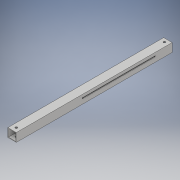
# Autodesk Inventor part: CLB_031_ScissorLiftBase19
Saved by Autodesk Inventor 2018.3 (Build 223284000, 284)
## iProperties
Created: 2020-01-24
Part Number: CLB_031_ScissorLiftBase19
Material: Generic
Document SubType Name: Modeling
Designer: Cooper
Density: 1 g/cm^3
Appearance: Default
Mass: 64.5264 g
Surface Area: 826.986 cm^2
Volume: 64.5264 cm^3
Author: Cooper
Autodesk Inventor part; units mm, degrees
ref_plane "YZ Plane" through (0, 0, 0) normal (1, 0, 0) x (0, 1, 0)
ref_plane "XZ Plane" through (0, 0, 0) normal (0, 1, 0) x (-1, 0, 0)
ref_plane "XY Plane" through (0, 0, 0) normal (0, 0, 1) x (1, 0, 0)
sketch "Sketch1" plane through (0, 0, 0) normal (0, 0, 1) x (1, 0, 0)
  line L0 (0, 0) -> (25.4, 0)
  line L1 (25.4, 0) -> (25.4, 25.4)
  line L2 (25.4, 25.4) -> (0, 25.4)
  line L3 (0, 25.4) -> (0, 0)
  line L4 (1.5875, 23.8125) -> (23.8125, 23.8125)
  line L5 (23.8125, 23.8125) -> (23.8125, 1.5875)
  line L6 (23.8125, 1.5875) -> (1.5875, 1.5875)
  line L7 (1.5875, 1.5875) -> (1.5875, 23.8125)
  dimension "d0" = 25.4
  dimension "d1" = 25.4
  dimension "d2" = 1.5875
  constraints: 16 end point, 4 parallel, 2 perpendicular, 1 horizontal, 3 other
  measures "d0" distance of L2.end L0.start
  measures "d1" distance of L0.start L0.end
  measures "d2" distance between parallel lines of L2 L4
extrude "Extrusion1" add sketch "Sketch1" along normal blind 508
sketch "Sketch2" plane through (0, 0, 0) normal (-1, 0, 0) x (0, 0, 1)
  line L0 (0, 25.4) -> (0, 0) projected
  line L1 (0, 0) -> (508, 0) projected
  line L2 (508, 25.4) -> (508, 0) projected
  line L3 (0, 25.4) -> (508, 25.4) projected
  line L4 (95.25, 16.8275) -> (311.15, 16.8275)
  arc A0 (311.15, 13.6525) -> (311.15, 16.8275) centre (311.15, 15.24) ccw
  line L5 (311.15, 13.6525) -> (95.25, 13.6525)
  arc A1 (95.25, 16.8275) -> (95.25, 13.6525) centre (95.25, 15.24) ccw
  dimension "d5" = 3.175
  dimension "d6" = 215.9
  dimension "d9" = 10.16
  dimension "d24" = 95.25
  constraints: 4 end point, 4 point on circle, 4 tangent, 2 centre point, 1 horizontal, 1 parallel
  measures "d5" distance between parallel lines of L5 L4
  measures "d6" distance of A0.centre A1.centre
  measures "d9" distance from line of L3 A1.centre
  measures "d24" distance from line of L0 A1.centre
extrude "Extrusion2" cut sketch "Sketch2" against normal through all contours L4 A0 L5 A1
sketch "Sketch3" plane through (0, 25.4, 0) normal (0, 1, 0) x (1, 0, 0)
  line L0 (25.4, 0) -> (0, 0) projected
  line L1 (0, 0) -> (0, -508) projected
  line L2 (25.4, -508) -> (0, -508) projected
  line L3 (25.4, 0) -> (25.4, -508) projected
  point P0 (0, 0)
  point P1 (12.7, -495.3)
  dimension "d13" = 12.7
  dimension "d14" = 12.7
  dimension "d23" = 12.7
  measures "d13" distance from line of L1 point (12.7, -495.3)
  measures "d14" distance from line of L3 point (12.7, -495.3)
  measures "d23" distance from line of L2 point (12.7, -495.3)
hole "Hole1" at (12.7, 25.4, 495.3) direction (0, -1, 0) diameter 6.35 end through all
sketch "Sketch4" plane through (0, 0, 0) normal (0, 0, -1) x (-1, 0, 0)
  line L0 (-35.9744, 31.9382) -> (12.1084, 31.9382)
  line L1 (12.1084, 31.9382) -> (12.1084, -6.8439)
  line L2 (12.1084, -6.8439) -> (-35.9744, -6.8439)
  line L3 (-35.9744, -6.8439) -> (-35.9744, 31.9382)
  point P0 (0, 0)
  constraints: 8 end point, 2 parallel, 1 horizontal, 1 perpendicular
extrude "Extrusion3" cut sketch "Sketch4" against normal blind 44.45
sketch "Sketch5" plane through (0, 0, 508) normal (0, -1, 0) x (1, 0, 0)
  line L0 (0, -463.55) -> (25.4, -463.55) projected
  line L1 (25.4, -463.55) -> (25.4, 0) projected
  point P0 (0, -508)
  point P1 (12.7, -453.39)
  dimension "d27" = 10.16
  dimension "d28" = 12.7
  measures "d27" distance from line of L0 point (12.7, -453.39)
  measures "d28" distance from line of L1 point (12.7, -453.39)
hole "Hole2" at (12.7, 0, 54.61) direction (0, 1, 0) diameter 6.35 end through all
equation "\"d13\" = d14"
body "Solid1"
